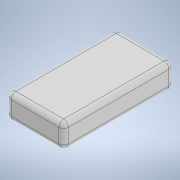
# Autodesk Inventor part: Battery
Saved by Autodesk Inventor 2021 (Build 250183000, 183)
## iProperties
Created: 2023-01-24
Part Number: Battery
Material: Genérico
Document SubType Name: Modeling
Designer: nicho
Density: 1 g/cm^3
Appearance: Padrão
Author: nicho
Autodesk Inventor part; units mm, degrees
ref_plane "YZ Plane" through (0, 0, 0) normal (1, 0, 0) x (0, 1, 0)
ref_plane "XZ Plane" through (0, 0, 0) normal (0, 1, 0) x (-1, 0, 0)
ref_plane "XY Plane" through (0, 0, 0) normal (0, 0, 1) x (1, 0, 0)
sketch "Esboço1" plane through (0, 0, 0) normal (0, 1, 0) x (-1, 0, 0)
  line L0 (-12, -23) -> (12, -23)
  line L1 (12, -23) -> (12, 23)
  line L2 (12, 23) -> (-12, 23)
  line L3 (-12, 23) -> (-12, -23)
  line L4 (-12, -23) -> (12, 23) construction
  line L5 (12, -23) -> (-12, 23) construction
  point P0 (0, 0)
  dimension "d0" = 24
  dimension "d1" = 46
  constraints: 12 end point, 2 midpoint, 2 parallel, 1 horizontal, 1 perpendicular
  measures "d0" distance of L2.end L1.end
  measures "d1" distance of L1.end L0.end
extrude "Extrusão1" add sketch "Esboço1" along normal blind 10
fillet "Arredondamento1" radius 2 12 edges at (12, 5, 23) (12, 10, 0) (0, 10, 23) (12, 0, 0) (12, 5, -23) (0, 0, 23) (-12, 5, 23) (0, 10, -23) (0, 0, -23) (-12, 5, -23) (-12, 0, 0) (-12, 10, 0)
